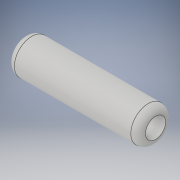
# Autodesk Inventor part: rubberhandlesleeve
Saved by Autodesk Inventor 2018 (Build 220112000, 112)
## iProperties
Created: 2019-01-10
Part Number: rubberhandlesleeve
Material: Generic
Document SubType Name: Modeling
Designer: This kid
Density: 1 g/cm^3
Appearance: Default
Author: This kid
Autodesk Inventor part; units mm, degrees
ref_plane "YZ Plane" through (0, 0, 0) normal (1, 0, 0) x (0, 1, 0)
ref_plane "XZ Plane" through (0, 0, 0) normal (0, 1, 0) x (-1, 0, 0)
ref_plane "XY Plane" through (0, 0, 0) normal (0, 0, 1) x (1, 0, 0)
sketch "Sketch2" plane through (0, 0, 0) normal (0, 0, 1) x (1, 0, 0)
  line L0 (99.6671, 2.919) -> (99.6671, -3.431)
  line L1 (99.6671, -3.431) -> (-13.8455, -3.431)
  line L2 (-13.8455, -3.431) -> (-13.8455, 2.919)
  line L3 (-9.8831, 2.919) -> (-9.8831, 9.269)
  line L4 (-9.8831, 9.269) -> (-13.8455, 9.269)
  line L5 (-13.8455, 9.269) -> (-13.8455, 2.919)
  line L6 (-9.8831, 2.919) -> (99.6671, 2.919)
  line L7 (-13.8455, 11.6503) -> (99.6671, 11.6503)
  point P0 (0, 0)
  dimension "d17" = 113.5126
  dimension "d18" = 6.35
  dimension "d19" = 3.9624
  dimension "d20" = 6.35
  dimension "d24" = 6.35
  dimension "d25" = 6.35
  dimension "d26" = 113.5126
  dimension "d27" = 2.3813
  constraints: 16 end point, 3 parallel, 2 horizontal, 1 perpendicular, 1 point on line, 1 other
  measures "d17" distance of L0.end L1.end
  measures "d18" distance of L0.start L0.end
  measures "d19" distance of L4.end L3.end
  measures "d20" distance of L3.end L3.start
  measures "d24" distance of L2.end L4.end
  measures "d25" distance of L2.end L1.end
  measures "d26" distance of L7.start L7.end
  measures "d27" distance of L7.start L4.end
revolve "Revolution1" add sketch "Sketch2" angle 360 about axis through (-13.8455, 11.6503, 0) along (1, 0, 0)
fillet "Fillet3" radius 6.35 2 edges at (99.6671, 26.7315, 0) (-13.8455, 26.7315, 0)
body "Solid3"
